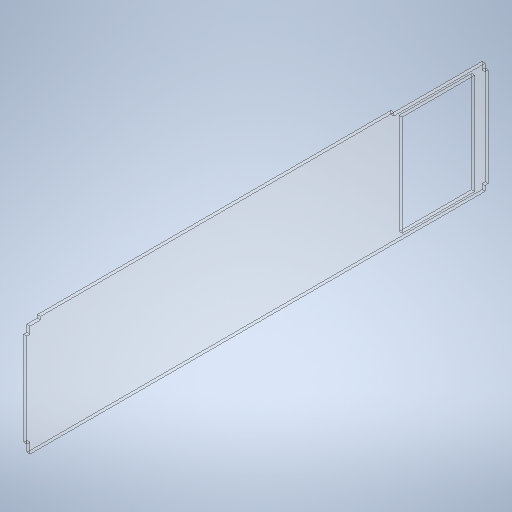
# Autodesk Inventor part: Lift cover of lifting
Saved by Autodesk Inventor 2025.4 (Build 294407000, 407)
## iProperties
Created: 2026-05-19
Part Number: Lift cover of lifting
Material: PMMA Plastic
Document SubType Name: Modeling
Designer: abdo2
Density: 1.188 g/cm^3
Appearance: Polycarbonate - Clear
Author: abdo2
Autodesk Inventor part; units mm, degrees
ref_plane "YZ Plane" through (0, 0, 0) normal (1, 0, 0) x (0, 1, 0)
ref_plane "XZ Plane" through (0, 0, 0) normal (0, 1, 0) x (-1, 0, 0)
ref_plane "XY Plane" through (0, 0, 0) normal (0, 0, 1) x (1, 0, 0)
sketch "Sketch1" plane through (0, 0, 0) normal (1, 0, 0) x (0, 1, 0)
  line L0 (0, 0) -> (442, 0)
  line L1 (442, 0) -> (442, -110)
  line L2 (442, -110) -> (0, -110)
  line L3 (0, -110) -> (0, 0)
  line L4 (3, 0) -> (3, -10)
  line L5 (3, -10) -> (0, -10)
  line L6 (3, -110) -> (3, -100)
  line L7 (3, -100) -> (0, -100)
  line L8 (13, 0) -> (13, -3)
  line L9 (13, -3) -> (3, -3)
  line L10 (442, -3) -> (354, -3)
  line L11 (354, -3) -> (354, 0)
  dimension "d0" = 442
  dimension "d1" = 110
  dimension "d2" = 3
  dimension "d3" = 10
  dimension "d4" = 10
  dimension "d5" = 10
  dimension "d6" = 3
  dimension "d7" = 88
  dimension "d8" = 3
  constraints: 24 end point, 10 point on line, 6 perpendicular, 3 parallel, 1 horizontal, 1 vertical
  measures "d0" distance of L1.end L2.end
  measures "d1" distance of L0.end L1.end
  measures "d2" distance between parallel lines of L3 L4
  measures "d3" distance between parallel lines of L0 L5
  measures "d4" distance between parallel lines of L2 L7
  measures "d5" distance of L8.end L9.end
  measures "d6" distance between parallel lines of L0 L9
  measures "d7" distance of L10.start L10.end
  measures "d8" distance between parallel lines of L0 L10
extrude "Extrusion1" add sketch "Sketch1" along normal blind 3 contours L5 L4 L9 L8 L0 L11 L10 L1 L2 L6 L7 L3
sketch "Sketch2" plane through (0, 442, -3) normal (0, 1, 0) x (1, 0, 0)
  line L0 (0, 7) -> (0, 97) projected
  line L1 (0, 7) -> (3, 7)
  line L2 (3, 7) -> (3, 97) projected
  line L3 (0, 7) -> (0, 102)
  line L4 (0, 97) -> (0, 107) projected
  line L5 (3, 97) -> (3, 107) projected
  line L6 (3, 102) -> (0, 102)
  line L7 (3, 102) -> (3, 7)
  line L8 (0, 7) -> (3, 7) projected
  line L9 (0, 107) -> (3, 107) projected
  line L10 (0, 0) -> (3, 0) projected
  point P0 (0, -3)
  point P1 (0, 97)
  dimension "d12" = 5
  dimension "d15" = 7
  constraints: 8 end point, 2 midpoint, 2 perpendicular, 2 point on line, 1 horizontal
  measures "d12" distance between parallel lines of L9 L6
  measures "d15" distance between parallel lines of L10 L1
extrude "Extrusion2" add sketch "Sketch2" along normal blind 3 contours L0 L3 L6 L5 L2 L1
sketch "Sketch3" plane through (3, 0, 0) normal (1, 0, 0) x (0, 0, -1)
  line L0 (8, 432) -> (8, 362)
  line L1 (8, 362) -> (105, 362)
  line L2 (105, 362) -> (105, 432)
  line L3 (105, 432) -> (8, 432)
  line L4 (3, 442) -> (3, 354) projected
  line L5 (110, 3) -> (110, 442) projected
  line L6 (10, 445) -> (105, 445) projected
  point P0 (0, 0)
  dimension "d16" = 5
  dimension "d17" = 5
  dimension "d18" = 70
  dimension "d19" = 13
  constraints: 8 end point, 3 perpendicular, 1 vertical
  measures "d16" distance between parallel lines of L4 L0
  measures "d17" distance between parallel lines of L5 L2
  measures "d18" distance between parallel lines of L1 L3
  measures "d19" distance between parallel lines of L6 L3
extrude "Extrusion3" cut sketch "Sketch3" against normal blind 3
body "Solid1"
